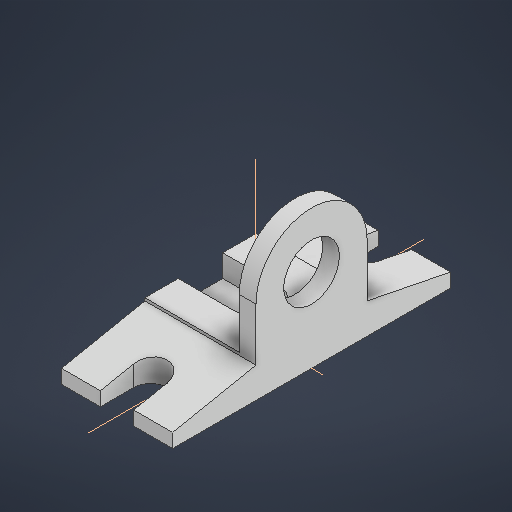
# Autodesk Inventor part: Pieza2
Saved by Autodesk Inventor 2026 (Build 300175000, 175)
## iProperties
Created: 2025-03-28
Part Number: Pieza2
Material: Genérico
Document SubType Name: Modeling
Designer: LabB305
Density: 1 g/cm^3
Appearance: Valor por defecto
Author: LabB305
Autodesk Inventor part; units mm, degrees
ref_plane "YZ Plane" through (0, 0, 0) normal (1, 0, 0) x (0, 1, 0)
ref_plane "XZ Plane" through (0, 0, 0) normal (0, 1, 0) x (-1, 0, 0)
ref_plane "XY Plane" through (0, 0, 0) normal (0, 0, 1) x (1, 0, 0)
sketch "Boceto1" plane through (0, 0, 0) normal (0, 1, 0) x (-1, 0, 0)
  line L0 (0, 0) -> (100, 0)
  line L1 (100, 0) -> (100, 250)
  line L2 (100, 250) -> (30, 250)
  line L3 (0, 0) -> (0, 190)
  circle A0 centre (0, 190) radius 30
  line L4 (30, 250) -> (30, 190)
  line L5 (0, 40) -> (100, 40)
  line L6 (-30, 190) -> (-30, 250)
  line L7 (-30, 250) -> (-100, 250)
  line L8 (-100, 250) -> (-100, 0)
  line L9 (-108.7956, 0) -> (-108.7956, 100)
  line L10 (-108.7956, 100) -> (100, 100)
  line L11 (100, 0) -> (100, -250)
  line L12 (100, -250) -> (30, -250)
  circle A1 centre (0, -190) radius 30
  line L13 (30, -250) -> (30, -190)
  line L14 (-30, -190) -> (-30, -250)
  line L15 (-30, -250) -> (-100, -250)
  line L16 (-100, -250) -> (-100, 0)
  point P0 (0, -40)
  point P1 (100, -40)
  point P2 (100, -100)
  dimension "d0" = 100
  dimension "d1" = 250
  dimension "d2" = 70
  dimension "d3" = 190
  dimension "d4" = 60
  dimension "d6" = 70
  dimension "d7" = 100
  constraints: 34 end point, 11 symmetric about line, 5 perpendicular, 5 point on line, 4 point on circle, 2 centre point, 2 coincident, 2 horizontal, 2 tangent, 2 vertical, 1 parallel, 1 other
  measures "d0" distance of L0.start L0.end
  measures "d1" distance of L0.end L1.end
  measures "d2" distance of L1.end L2.end
  measures "d3" distance of L0.start L3.end
  measures "d4" diameter of A0
  measures "d6" distance of L6.end L7.end
  measures "d7" distance of L9.start L9.end
extrude "Extrusión1" add sketch "Boceto1" along normal blind 25 contours L3 L5 L1 L0 | L0 L11 L12 L13 A1 L14 L15 L16 L8 L10 L3 | L3 L10 L1 L5 | L10 L8 L7 L6 A0 L3 | L3 A0 L4 L2 L1 L10
sketch "Boceto2" plane through (0, 25, 0) normal (0, 1, 0) x (1, 0, 0)
  circle A0 centre (0, 0) radius 40
  line L0 (100, -250) -> (100, 250) projected
  line L1 (100, 0) -> (100, -100)
  line L2 (100, -100) -> (-100, -100)
  line L3 (-100, 250) -> (-100, -250) projected
  line L4 (-40, 0) -> (40, 0)
  line L5 (100, 100) -> (-100, 100)
  line L6 (0, -40) -> (-100, -40)
  line L7 (0, 40) -> (-100, 40)
  dimension "d10" = 80
  dimension "d11" = 100
  constraints: 12 end point, 4 point on circle, 4 point on line, 3 perpendicular, 2 symmetric about line, 2 tangent, 1 centre point, 1 coincident, 1 horizontal, 1 midpoint
  measures "d10" diameter of A0
  measures "d11" distance of L1.start L1.end
extrude "Extrusión2" add sketch "Boceto2" along normal blind 35 contours A0 L7 L3 L5 L0 L2 L6
sketch "Boceto3" plane through (0, 25, 0) normal (0, 1, 0) x (1, 0, 0)
  line L0 (-100, 40) -> (0, 40) projected
  circle A0 centre (0, 0) radius 40
  line L1 (0, 40) -> (-100, 40)
  line L2 (0, -40) -> (-100, -40)
  line L3 (-100, 40) -> (-100, -40) projected
  line L4 (-100, 40) -> (-100, -40)
  constraints: 6 end point, 3 equal length, 2 point on circle, 2 tangent, 1 centre point, 1 coincident
extrude "Extrusión3" cut sketch "Boceto3" against normal blind 5
sketch "Boceto4" plane through (0, 60, 0) normal (0, 1, 0) x (1, 0, 0)
  line L0 (100, 100) -> (-100, 100) projected
  line L1 (100, -100) -> (-100, -100) projected
  line L2 (100, 100) -> (70, 100)
  line L3 (70, 100) -> (70, -100)
  line L4 (70, -100) -> (100, -100)
  line L5 (100, -100) -> (100, 100)
  point P0 (0, 0)
  dimension "d16" = 30
  constraints: 8 end point, 2 parallel, 1 horizontal, 1 perpendicular, 1 point on line
  measures "d16" distance of L4.end L3.end
extrude "Extrusión4" add sketch "Boceto4" along normal blind 190
sketch "Boceto5" plane through (70, 60, -100) normal (-1, 0, 0) x (0, 0, 1)
  line L0 (200, 0) -> (0, 0) projected
  line L1 (100, 0) -> (100, 90)
  circle A0 centre (100, 90) radius 50
  point P0 (100, -60)
  dimension "d19" = 90
  dimension "d20" = 100
  constraints: 2 end point, 1 centre point, 1 coincident, 1 midpoint, 1 vertical
  measures "d19" distance of L1.start L1.end
  measures "d20" diameter of A0
extrude "Extrusión5" cut sketch "Boceto5" against normal blind 190
fillet "Empalme1" radius 100 2 edges at (85, 250, -100) (85, 250, 100)
sketch "Boceto6" plane through (-100, 0, -250) normal (-1, 0, 0) x (0, 0, 1)
  line L0 (150, 25) -> (150, 60) projected
  line L1 (150, 60) -> (150, 55)
  line L2 (150, 25) -> (0, 25) projected
  line L3 (150, 55) -> (0, 25)
  line L4 (250, 88.3729) -> (250, -17.9249)
  line L5 (350, 25) -> (350, 60)
  line L6 (350, 25) -> (500, 25)
  line L7 (350, 55) -> (500, 25)
  point P0 (250, 0)
  dimension "d24" = 5
  constraints: 12 end point, 4 symmetric about line, 2 point on line, 1 vertical
  measures "d24" distance of L0.end L1.end
extrude "Extrusión6" add sketch "Boceto6" against normal blind 200
sketch "Boceto7" plane through (0, 25, -190) normal (0, -1, 0) x (1, 0, 0)
  line L0 (30, -60) -> (30, 0) projected
  circle A0 centre (0, 0) radius 30
  line L1 (30, 0) -> (30, -60)
  line L2 (-30, -60) -> (30, -60) projected
  line L3 (-30, -60) -> (-100, -60) projected
  line L4 (30, -60) -> (-30, -60)
  line L5 (-30, -60) -> (-30, 0)
  line L6 (105.1195, 190) -> (-118.3663, 190)
  line L7 (30, 440) -> (30, 380)
  circle A1 centre (0, 380) radius 30
  line L8 (-30, 440) -> (30, 440)
  line L9 (-30, 440) -> (-30, 380)
  point P0 (0, 190)
  constraints: 14 end point, 5 point on circle, 5 symmetric about line, 2 centre point, 2 horizontal, 1 collinear, 1 perpendicular, 1 other
extrude "Extrusión7" cut sketch "Boceto7" against normal blind 200
